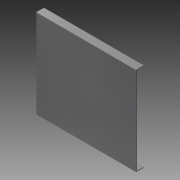
# Autodesk Inventor part: controller_table
Saved by Autodesk Inventor 2015 (Build 190159000, 159)
## iProperties
Created: 2015-12-24
Part Number: controller_table
Material: ステンレス鋼
Document SubType Name: Modeling
Designer: Ryo
Density: 8 g/cm^3
Appearance: 半つや出し
Author: Ryo
Autodesk Inventor part; units mm, degrees
ref_plane "YZ Plane" through (0, 0, 0) normal (1, 0, 0) x (0, 1, 0)
ref_plane "XZ Plane" through (0, 0, 0) normal (0, 1, 0) x (-1, 0, 0)
ref_plane "XY Plane" through (0, 0, 0) normal (0, 0, 1) x (1, 0, 0)
sketch "スケッチ1" plane through (0, 0, 0) normal (0, 1, 0) x (-1, 0, 0)
  line L0 (-290, 257.5) -> (290, 257.5)
  line L1 (290, 257.5) -> (290, -257.5)
  line L2 (290, -257.5) -> (-290, -257.5)
  line L3 (-290, -257.5) -> (-290, 257.5)
  line L4 (-290, 257.5) -> (290, -257.5) construction
  line L5 (290, 257.5) -> (-290, -257.5) construction
  line L6 (285, 257.5) -> (285, -257.5)
  line L7 (290, -252.5) -> (-290, -252.5)
  line L8 (290, 252.5) -> (-290, 252.5)
  point P0 (0, 0)
  dimension "d0" = 580
  dimension "d1" = 515
  dimension "d2" = 5
  dimension "d3" = 5
  dimension "d4" = 5
  constraints: 18 end point, 6 point on line, 4 perpendicular, 2 midpoint, 2 parallel, 1 horizontal
  measures "d0" distance of L1.end L2.end
  measures "d1" distance of L0.end L1.end
  measures "d2" distance between parallel lines of L6 L1
  measures "d3" distance between parallel lines of L2 L7
  measures "d4" distance between parallel lines of L0 L8
extrude "押し出し1" add sketch "スケッチ1" along normal blind 45 contours L0 L6 L8 L3 | L0 L1 L8 L6 | L7 L6 L2 L3 | L7 L1 L2 L6
extrude "押し出し2" add sketch "スケッチ1" along normal blind 5 contours L0 L6 L8 L3 | L8 L6 L7 L3 | L7 L6 L2 L3
fillet "フィレット1" radius 2.5 1 edges at (0, 0, -257.5)
fillet "フィレット2" radius 2.5 1 edges at (0, 0, 257.5)
extrude "押し出し3" add sketch "スケッチ1" along normal blind 5 contours L8 L6 L7 L3 | L8 L1 L7 L6
